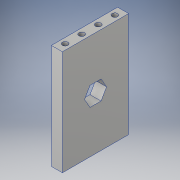
# Autodesk Inventor part: Pivot Plate
Saved by Autodesk Inventor 2019.4 (Build 234330000, 330)
## iProperties
Created: 2020-01-06
Part Number: Pivot Plate
Material: Aluminum 6061
Document SubType Name: Modeling
Designer: admin
Density: 2.7 g/cm^3
Appearance: Aluminum - Flat
Mass: 204.151 g
Surface Area: 253.384 cm^2
Volume: 75.6114 cm^3
Author: admin
Autodesk Inventor part; units mm, degrees
ref_plane "YZ Plane" through (0, 0, 0) normal (1, 0, 0) x (0, 1, 0)
ref_plane "XZ Plane" through (0, 0, 0) normal (0, 1, 0) x (-1, 0, 0)
ref_plane "XY Plane" through (0, 0, 0) normal (0, 0, 1) x (1, 0, 0)
sketch "Sketch1" plane through (0, 0, 0) normal (1, 0, 0) x (0, 1, 0)
  line L0 (-47.5, 30) -> (47.5, 30)
  line L1 (47.5, 30) -> (47.5, -30)
  line L2 (47.5, -30) -> (-47.5, -30)
  line L3 (-47.5, -30) -> (-47.5, 30)
  line L4 (-47.5, 30) -> (47.5, -30) construction
  line L5 (47.5, 30) -> (-47.5, -30) construction
  point P0 (0, 0)
  dimension "d0" = 95
  dimension "d1" = 60
  constraints: 12 end point, 2 midpoint, 2 parallel, 1 horizontal, 1 perpendicular
  measures "d0" distance of L1.end L2.end
  measures "d1" distance of L0.end L1.end
extrude "Extrusion1" add sketch "Sketch1" along normal mid plane 10
sketch "Sketch2" plane through (-5, 47.5, 30) normal (0, 1, 0) x (1, 0, 0)
  circle A0 centre (5, 52.5) radius 2.5
  circle A1 centre (5, 37.5) radius 2.5
  circle A2 centre (5, 22.5) radius 2.5
  circle A3 centre (5, 7.5) radius 2.5
  circle A4 centre (5, -7.5) radius 2.5
  line L0 (10, 60) -> (0, 60) projected
  line L1 (10, 60) -> (10, 0) projected
  point P0 (5, 30)
  dimension "d4" = 5
  dimension "d5" = 5
  dimension "d6" = 5
  dimension "d7" = 5
  dimension "d9" = 15
  dimension "d10" = 15
  dimension "d11" = 15
  dimension "d12" = 5
  dimension "d13" = 15
  dimension "d14" = 7.5
  dimension "d15" = 5
  dimension "d16" = 5
  dimension "d17" = 5
  dimension "d18" = 5
  dimension "d19" = 5
  constraints: 5 centre point
  measures "d4" diameter of A0
  measures "d5" diameter of A1
  measures "d6" diameter of A2
  measures "d7" diameter of A3
  measures "d9" distance of A2.centre A1.centre
  measures "d10" distance of A3.centre A2.centre
  measures "d11" distance of A0.centre A1.centre
  measures "d12" diameter of A4
  measures "d13" distance of A3.centre A4.centre
  measures "d14" distance from line of L0 A0.centre
  measures "d15" distance from line of L1 A4.centre
  measures "d16" distance from line of L1 A3.centre
  measures "d17" distance from line of L1 A2.centre
  measures "d18" distance from line of L1 A1.centre
  measures "d19" distance from line of L1 A0.centre
extrude "Extrusion2" cut sketch "Sketch2" against normal blind 20
sketch "Sketch3" plane through (5, 0, 0) normal (1, 0, 0) x (0, 0, -1)
  line L0 (-30, 47.5) -> (-30, -47.5) projected
  line L1 (-30, -47.5) -> (30, -47.5) projected
  line L2 (30, -47.5) -> (30, 47.5) projected
  line L3 (30, 47.5) -> (-30, 47.5) projected
  circle A0 centre (0, 0) radius 10 construction
  line L4 (10, 0) -> (5, -8.6603)
  line L5 (5, -8.6603) -> (-5, -8.6603)
  line L6 (-5, -8.6603) -> (-10, 0)
  line L7 (-10, 0) -> (-5, 8.6603)
  line L8 (-5, 8.6603) -> (5, 8.6603)
  line L9 (5, 8.6603) -> (10, 0)
  line L10 (30, 47.5) -> (-30, 47.5) projected
  line L11 (0, 47.5) -> (0, 0) construction
  line L12 (0, 0) -> (30, 0) construction
  line L13 (30, -47.5) -> (30, 47.5) projected
  dimension "d30" = 20
  constraints: 16 end point, 2 midpoint, 2 perpendicular, 1 coincident, 1 horizontal, 1 horizontal alignment, 15 other
extrude "Extrusion3" cut sketch "Sketch3" against normal through all contours L4 L5 L6 L7 L8 L9
mirror "Mirror1" about plane through (0, 0, 0) normal (0, 1, 0) of "Extrusion2"
body "Solid1"
